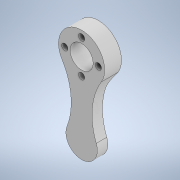
# Autodesk Inventor part: arm_linkage_1
Saved by Autodesk Inventor 2020 (Build 240168000, 168)
## iProperties
Created: 2019-10-19
Part Number: arm_linkage_1
Material: Generic
Document SubType Name: Modeling
Designer: psrob
Density: 1 g/cm^3
Appearance: Default
Author: psrob
Autodesk Inventor part; units mm, degrees
ref_plane "YZ Plane" through (0, 0, 0) normal (1, 0, 0) x (0, 1, 0)
ref_plane "XZ Plane" through (0, 0, 0) normal (0, 1, 0) x (-1, 0, 0)
ref_plane "XY Plane" through (0, 0, 0) normal (0, 0, 1) x (1, 0, 0)
sketch "Sketch1" plane through (0, 0, 0) normal (0, 0, 1) x (1, 0, 0)
  circle A0 centre (0, 0) radius 11 projected
  circle A1 centre (0, 0) radius 5 projected
  circle A2 centre (-8, 0) radius 1.5 projected
  circle A3 centre (0, 8) radius 1.5 projected
  circle A4 centre (8, 0) radius 1.5 projected
  circle A5 centre (0, -8) radius 1.5 projected
  circle A6 centre (0, 0) radius 6
  circle A7 centre (0, 0) radius 11
  point P0 (0, 0)
  dimension "d0" = 12
  dimension "d1" = 22
  constraints: 2 centre point, 2 coincident
  measures "d0" diameter of A6
  measures "d1" diameter of A7
extrude "Extrusion1" add sketch "Sketch1" along normal blind 8 contours A0
thicken "Thicken1" operation add thickness 0.5 both sides no extend neighbours yes toward (-0.9967573, 0.0804666, 0) faces at (5.9805, -0.4828, 5.3333)
sketch "Sketch2" plane through (0, 0, 8) normal (0, 0, 1) x (1, 0, 0)
  circle A0 centre (0, 0) radius 11 projected
  circle A1 centre (-8, 0) radius 1.5 projected
  circle A2 centre (0, -8) radius 1.5 projected
  circle A3 centre (0, 0) radius 5.5 projected
  circle A4 centre (8, 0) radius 1.5 projected
  circle A5 centre (0, 8) radius 1.5 projected
  line L0 (0, 0) -> (0, -35)
  circle A6 centre (0, -35) radius 7.5
  line L1 (0, 0) -> (-9.3786, -5.7482)
  line L2 (0, -35) -> (-6.9913, -32.285)
  line L3 (0, -35) -> (6.9913, -32.285)
  line L4 (0, 0) -> (9.3786, -5.7482)
  circle A7 centre (0, 0) radius 11 projected
  arc A8 (-6.9913, -32.285) -> (-9.3786, -5.7482) centre (-34.9567, -21.425) ccw
  arc A9 (9.3786, -5.7482) -> (6.9913, -32.285) centre (34.9567, -21.425) ccw
  point P0 (0, 0)
  dimension "d6" = 35
  dimension "d7" = 15
  dimension "d8" = 30
  dimension "d9" = 30
  constraints: 10 end point, 7 point on circle, 4 line through centre, 3 centre point, 1 coincident, 1 vertical, 2 other
  measures "d6" distance of L0.start L0.end
  measures "d7" diameter of A6
  measures "d8" radius of A8
  measures "d9" radius of A9
extrude "Extrusion2" add sketch "Sketch2" against normal blind 5 contours A0 L0 A6 A8 | A9 A6 L0 A0 | L2 L3 A6 | A6 L0 L2 | L3 L0 A6
fillet "Fillet1" radius 3 1 edges at (0, -11, 3)
body "Solid1"
